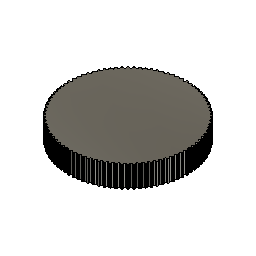
gear_88z (Autodesk Fusion 360 design; units mm, degrees)
Autodesk Fusion 360 part; units mm, degrees
sketch "Sketch1" plane through (0, 0, 0) normal (0, 0, 1) x (1, 0, 0) in component "gt2 pulley"
  circle A0 centre (0, 0) radius 28.0113 construction
  circle A1 centre (0, 0) radius 27.0073 construction
  line L0 (0, 0) -> (0, 28.0113) construction
  line L1 (0, 0) -> (0.9998, 27.9934) construction
  line L2 (0, 0) -> (1.4045, 27.976) construction
  circle A2 centre (0, 0) radius 27.7573 construction
  arc A3 (0.3969, 27.6213) -> (0.4749, 27.3231) centre (1.3918, 27.7224) ccw
  circle A4 centre (0, 0) radius 27.6073 construction
  arc A5 (0.2489, 27.7562) -> (0, 27.7573) centre (0, 0) ccw
  arc A6 (0.3969, 27.6213) -> (0.2489, 27.7562) centre (0.2476, 27.6062) ccw
  arc A7 (0.4749, 27.3231) -> (0.964, 26.9901) centre (0.9838, 27.5447) ccw
  arc A8 (0, 27.7573) -> (-0.2489, 27.7562) centre (0, 0) ccw
  arc A9 (-0.2489, 27.7562) -> (-0.3969, 27.6213) centre (-0.2476, 27.6062) ccw
  arc A10 (-0.4749, 27.3231) -> (-0.3969, 27.6213) centre (-1.3918, 27.7224) ccw
  arc A11 (-0.9638, 26.9901) -> (-0.4749, 27.3231) centre (-0.9838, 27.5447) ccw
  arc A12 (0.964, 26.9901) -> (-0.964, 26.9901) centre (0, 0) ccw
  point P0 (1.3918, 27.7224)
  point P1 (0, 27.7573)
  dimension "d18" = 56.0225
  dimension "d19" = 2.045
  dimension "d22" = 1.004
  dimension "d24" = 0.75
  dimension "d26" = 1
  dimension "d27" = 0.15
  dimension "d28" = 0.15
  dimension "d47" = 0.555
  dimension "d52" = 3.812
  constraint coincident A0.centre A1.centre
  constraint coincident A0 L0.end
  constraint vertical L0
  constraint coincident A0 L1.end
  constraint coincident A0 L2.end
  constraint concentric A1 A2
  constraint coincident A1 A7.end
  constraint coincident L1 A7.end
  constraint coincident A2 P0
  constraint coincident L2 P0
  constraint coincident P0 A3.centre
  constraint coincident A2 P1
  constraint coincident L0 P1
  constraint concentric A2 A4
  constraint coincident P1 A5.end
  constraint coincident A4 A6.centre
  constraint coincident A3.start A6.start
  constraint tangent A3 A6
  constraint tangent A3 A7
  constraint symmetric L0 A7.end A12.end
  constraint symmetric L0 A3.start A9.end
  constraint symmetric L0 A3.end A10.start
  constraint symmetric L0 A3 A10
  constraint symmetric L0 A5.start A8.end
  constraint symmetric L0 P1 A5.end
  constraint symmetric L0 A5 A8
  constraint symmetric L0 A6 A9
  constraint symmetric L0 A7 A11
  constraint coincident A1 A11.start
  constraint tangent A1 A7
  constraint coincident L1 A7.centre
  measures "d18" diameter of A0
  measures "d19" angle of L0 L1
  measures "d22" distance of A0 A1
  measures "d24" distance of A1 A2
  measures "d26" radius of A3
  measures "d27" distance of A2 A4
  measures "d28" radius of A6
  measures "d47" radius of A7
extrude "Extrude1" add sketch "Sketch1" along normal blind 10 makes body 1
pattern_circular "C-Pattern1" count 88 over 360 about axis through (0, 0, 1.75) along (0, 0, 1) of bodies 1 makes body 2 at (-2.4605, 26.895, 3.3333) makes body 3 at (-4.5841, 26.6154, 6.6667) makes body 4 at (-5.0059, 26.5393, 3.3333) makes body 5 at (-8.3252, 25.6921, 6.6667) makes body 6 at (-8.7319, 25.5567, 3.3333) makes body 7 at (-11.3165, 24.522, 6.6667) makes body 8 at (-13.5962, 23.3353, 6.6667) makes body 9 at (-14.6912, 22.6619, 6.6667) makes body 10 at (-16.7788, 21.1628, 6.6667) makes body 11 at (-18.2458, 19.9119, 6.6667) makes body 12 at (-19.4719, 18.7146, 6.6667) makes body 13 at (-20.4807, 17.6049, 6.6667) makes body 14 at (-21.6844, 16.099, 6.6667) makes body 15 at (-22.7777, 14.511, 6.6667) makes body 16 at (-24.0539, 12.2802, 6.6667) makes body 17 at (-24.611, 11.1217, 6.6667) makes body 18 at (-25.3417, 9.3377, 6.6667) makes body 19 at (-26.0591, 7.0935, 6.6667) makes body 20 at (-26.4987, 5.2164, 6.6667) makes body 21 at (-26.7474, 3.7375, 6.6667) makes body 22 at (-26.9816, 1.1781, 6.6667) makes body 23 at (-26.9969, -0.7497, 6.6667) makes body 24 at (-26.8746, -2.6737, 6.6667) makes body 25 at (-26.6154, -4.5841, 6.6667) makes body 26 at (-26.2205, -6.4712, 6.6667) makes body 27 at (-26.1145, -6.8865, 3.3333) makes body 28 at (-25.5567, -8.7319, 3.3333) makes body 29 at (-24.522, -11.3165, 6.6667) makes body 30 at (-23.3353, -13.5962, 6.6667) makes body 31 at (-22.3059, -15.2263, 6.6667) makes body 32 at (-21.1628, -16.7788, 6.6667) makes body 33 at (-19.9119, -18.2458, 6.6667) makes body 34 at (-18.7146, -19.4719, 6.6667) makes body 35 at (-17.6049, -20.4807, 6.6667) makes body 36 at (-15.5784, -22.0614, 6.6667) makes body 37 at (-15.2264, -22.3058, 3.3333) makes body 38 at (-12.2802, -24.0539, 6.6667) makes body 39 at (-10.5329, -24.8686, 6.6667) makes body 40 at (-10.137, -25.0327, 3.3333) makes body 41 at (-7.0935, -26.0591, 6.6667) makes body 42 at (-6.4713, -26.2205, 3.3333) makes body 43 at (-3.1, -26.8288, 6.6667) makes body 44 at (-1.1781, -26.9816, 6.6667) makes body 45 at (-0.7498, -26.9969, 3.3333) makes body 46 at (2.6737, -26.8746, 6.6667) makes body 47 at (4.5841, -26.6154, 6.6667) makes body 48 at (5.0059, -26.5393, 3.3333) makes body 49 at (6.8865, -26.1145, 3.3333) makes body 50 at (8.7319, -25.5567, 3.3333) makes body 51 at (10.5328, -24.8687, 3.3333) makes body 52 at (13.0371, -23.6522, 6.6667) makes body 53 at (14.6912, -22.6619, 6.6667) makes body 54 at (16.7788, -21.1628, 6.6667) makes body 55 at (18.2458, -19.9119, 6.6667) makes body 56 at (19.4719, -18.7146, 6.6667) makes body 57 at (20.4807, -17.6049, 6.6667) makes body 58 at (21.6844, -16.099, 6.6667) makes body 59 at (22.3058, -15.2264, 3.3333) makes body 60 at (24.0539, -12.2802, 6.6667) makes body 61 at (24.8686, -10.5329, 6.6667) makes body 62 at (25.5567, -8.732, 6.6667) makes body 63 at (25.9432, -7.506, 6.6667) makes body 64 at (26.4126, -5.6361, 6.6667) makes body 65 at (26.7474, -3.7375, 6.6667) makes body 66 at (26.9816, -1.1781, 6.6667) makes body 67 at (26.9969, -0.7498, 3.3333) makes body 68 at (26.8746, 2.6737, 6.6667) makes body 69 at (26.6154, 4.5841, 6.6667) makes body 70 at (26.3671, 5.8454, 6.6667) makes body 71 at (26.1145, 6.8865, 3.3333) makes body 72 at (25.5567, 8.7319, 3.3333) makes body 73 at (24.2458, 11.8969, 6.6667) makes body 74 at (23.3353, 13.5962, 6.6667) makes body 75 at (22.6619, 14.6912, 6.6667) makes body 76 at (21.1628, 16.7788, 6.6667) makes body 77 at (19.9119, 18.2458, 6.6667) makes body 78 at (18.7146, 19.4719, 6.6667) makes body 79 at (17.1126, 20.8938, 6.6667) makes body 80 at (16.099, 21.6844, 6.6667) makes body 81 at (15.2264, 22.3058, 3.3333) makes body 82 at (12.2802, 24.0539, 6.6667) makes body 83 at (11.1217, 24.611, 6.6667) makes body 84 at (9.3377, 25.3417, 6.6667) makes body 85 at (6.8866, 26.1145, 3.3333) makes body 86 at (5.2164, 26.4987, 6.6667) makes body 87 at (3.1, 26.8288, 6.6667) makes body 88 at (1.8199, 26.9459, 6.6667)
sketch "Sketch2" plane through (0, 0, 10) normal (0, 0, 1) x (-1, 0, 0)
  arc A0 (-10.0245, -25.7411) -> (-9.933, -25.9191) centre (-9.8794, -25.779) ccw
  arc A1 (-9.933, -25.9191) -> (-9.4665, -26.0931) centre (0, 0) ccw
  arc A2 (-9.4665, -26.0931) -> (-9.2808, -26.0185) centre (-9.4153, -25.9521) ccw
  arc A3 (-9.1035, -25.7664) -> (-9.2808, -26.0185) centre (-8.384, -26.4608) ccw
  arc A4 (-8.529, -25.6252) -> (-9.1035, -25.7664) centre (-8.7042, -26.1518) ccw
  arc A5 (-10.3352, -24.9515) -> (-8.529, -25.6252) centre (0, 0) ccw
  arc A6 (-9.9934, -25.4345) -> (-10.3352, -24.9515) centre (-10.5476, -25.4642) ccw
  arc A7 (-10.0245, -25.7411) -> (-9.9934, -25.4345) centre (-10.992, -25.4881) ccw
  circle A8 centre (0, 0) radius 27.0073
  constraint concentric A1 A8
extrude "Extrude2" add sketch "Sketch2" against normal blind 10 contours A5 A8 bodies 1 2 3 4 5 6 7 8 9 10 11 12 13 14 15 16 17 18 19 20 21 22 23 24 25 26 27 28 29 30 31 32 33 34 35 36 37 38 39 40 41 42 43 44 45 46 47 48 49 50 51 52 53 54 55 56 57 58 59 60 61 62 63 64 65 66 67 68 69 70 71 72 73 74 75 76 77 78 79 80 81 82 83 84 85 86 87 88
extrude "Extrude4" [suppressed] in component "gt2 pulley"
pattern_circular "C-Pattern7" [suppressed] in component "gt2 pulley"
extrude "Extrude3" [suppressed] in component "gt2 pulley"
pattern_circular "C-Pattern6" [suppressed] in component "gt2 pulley"
extrude "Extrude2'" [suppressed] in component "gt2 pulley"
pattern_circular "C-Pattern5" [suppressed] in component "gt2 pulley"
extrude "Extrude1'" [suppressed] in component "gt2 pulley"
pattern_circular "C-Pattern4" [suppressed] in component "gt2 pulley"
pattern_circular "C-Pattern3" [suppressed] in component "gt2 pulley"
pattern_circular "C-Pattern2" [suppressed] in component "gt2 pulley"
pattern_circular "C-Pattern1'" [suppressed] in component "gt2 pulley"
copy_body "Body->Comp1" [suppressed] in component "Component"
copy_body "Body->Comp2" [suppressed] in component "Component'"
copy_body "Body->Comp3" [suppressed] in component "Component''"
copy_body "Body->Comp4" [suppressed] in component "Component'''"
copy_body "Body->Comp5" [suppressed] in component "Component''''"
copy_body "Body->Comp6" [suppressed] in component "Component'''''"
copy_body "Body->Comp7" [suppressed] in component "Component''''''"
copy_body "Body->Comp8" [suppressed] in component "Component'''''''"
copy_body "Body->Comp9" [suppressed] in component "Component''''''''"
copy_body "Body->Comp10" [suppressed] in component "Component'''''''''"
copy_body "Body->Comp11" [suppressed] in component "Component''''''''''"
copy_body "Body->Comp12" [suppressed] in component "Component'''''''''''"
copy_body "Body->Comp13" [suppressed] in component "Component''''''''''''"
copy_body "Body->Comp14" [suppressed] in component "Component'''''''''''''"
copy_body "Body->Comp15" [suppressed] in component "Component''''''''''''''"
copy_body "Body->Comp16" [suppressed] in component "Component'''''''''''''''"
copy_body "Body->Comp17" [suppressed] in component "Component''''''''''''''''"
copy_body "Body->Comp18" [suppressed] in component "Component'''''''''''''''''"
copy_body "Body->Comp19" [suppressed] in component "Component''''''''''''''''''"
copy_body "Body->Comp20" [suppressed] in component "Component'''''''''''''''''''"
component "gt2 pulley" placed x (1, 0, 0) y (0, 1, 0) z (0, 0, 1) at (0, 0, 0)
equation "NumTeeth = 88" comment "min 20"
equation "ToothPitch = 2 mm"
equation "PullyDia = NumTeeth * ToothPitch / PI"
equation "ToothAng = ( ( 360 / NumTeeth ) * 1 deg )"
equation "TransOffsetAngle = ToothAng * 0.2"
equation "Sholulder_Radius = 0.15 mm"
equation "Root_Radius = 0.555 mm"
equation "TransRadius = 1 mm"
equation "ToolHeight = 0.75 mm"
equation "PLD = 0.254 mm"
equation "d18 = PullyDia"
equation "d19 = ToothAng / 2"
equation "d22 = PLD + ToolHeight"
equation "d24 = ToolHeight"
equation "d26 = TransRadius"
equation "d27 = Sholulder_Radius"
equation "d31 = NumTeeth"
equation "d33 = NumTeeth"
equation "d35 = NumTeeth"
equation "d37 = NumTeeth"
equation "d41 = NumTeeth"
equation "d45 = NumTeeth"
equation "d47 = Root_Radius"
equation "d50 = NumTeeth"
